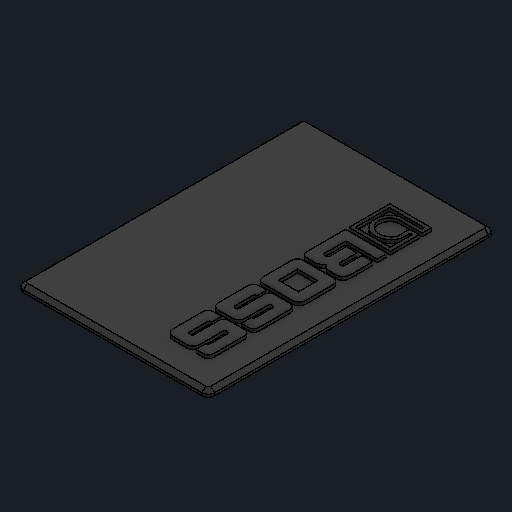
# Autodesk Inventor part: Pad
Saved by Autodesk Inventor 2026.2 (Build 302298000, 298)
## iProperties
Created: 2015-05-06
Part Number: Pad
Material: Rubber
Document SubType Name: Modeling
Designer: Philip
Density: 0.93 g/cm^3
Appearance: Rubber - Black
Author: Philip
Autodesk Inventor part; units mm, degrees
(part 1 of 2)
ref_plane "YZ Plane" through (0, 0, 0) normal (1, 0, 0) x (0, 1, 0)
ref_plane "XZ Plane" through (0, 0, 0) normal (0, 1, 0) x (-1, 0, 0)
ref_plane "XY Plane" through (0, 0, 0) normal (0, 0, 1) x (1, 0, 0)
sketch "Sketch1" plane through (0, 0, 0) normal (0, 1, 0) x (-1, 0, 0)
  line L0 (-19.05, 28.575) -> (19.05, 28.575)
  line L1 (19.05, 28.575) -> (19.05, -28.575)
  line L2 (19.05, -28.575) -> (-19.05, -28.575)
  line L3 (-19.05, -28.575) -> (-19.05, 28.575)
  point P0 (0, 0)
  dimension "d0" = 57.15
  dimension "d1" = 38.1
  dimension "d2" = 28.575
  dimension "d3" = 19.05
  constraints: 8 end point, 2 parallel, 1 horizontal, 1 perpendicular
  measures "d0" distance of L2.end L0.start
  measures "d1" distance of L1.end L2.end
  measures "d2" distance from line of L2 point (0, 0)
  measures "d3" distance from line of L1 point (0, 0)
extrude "Extrusion1" add sketch "Sketch1" along normal blind 1.27
fillet "Fillet1" radius 1.27 2 edges at (19.05, 0.635, 28.575) (-19.05, 0.635, 28.575)
fillet "Fillet1" radius 1.27 2 edges at (19.05, 0.635, -28.575) (-19.05, 0.635, -28.575)
chamfer "Chamfer1" distance 0.762 angle 45 8 edges at (19.05, 1.27, 0) (18.678, 1.27, -28.203) (0, 1.27, -28.575) (-18.678, 1.27, -28.203) (-19.05, 1.27, 0) (-18.678, 1.27, 28.203) (0, 1.27, 28.575) (18.678, 1.27, 28.203)
sketch "Sketch2" plane through (0, 1.27, 0) normal (0, 1, 0) x (1, 0, 0)
  spline S0 degree 3 poles (9.3958, 4.5889) (10.1252, 3.8936) (10.2655, 3.812) (10.8634, 3.789) (11.2905, 3.7727) (11.7187, 3.7634) (12.1459, 3.7736) (13.0489, 3.7954) (13.5879, 4.3543) (13.5894, 5.258) (13.5915, 6.5998) (13.5905, 7.9416) (13.5889, 9.2834) (13.5888, 9.4117) (13.575, 9.5399) (13.567, 9.6778) (12.8489, 9.6778) (12.163, 9.6778) (11.4348, 9.6778) (11.4348, 9.5086) (11.4348, 9.3648) (11.4348, 9.221) (11.4347, 8.2774) (11.4161, 7.3331) (11.443, 6.3902) (11.4552, 5.9625) (11.2394, 5.916) (10.901, 5.9027) (10.5127, 5.8874) (10.4743, 6.0999) (10.4779, 6.4041) (10.4876, 7.2297) (10.4812, 8.0555) (10.4812, 8.8813) (10.4812, 9.1406) (10.4812, 9.3999) (10.4812, 9.6605) (9.7415, 9.6605) (9.0682, 9.6605) (8.3475, 9.6605) (8.3475, 9.4797) (8.3475, 9.3219) (8.3475, 9.1641) (8.3475, 8.2647) (8.335, 7.3649) (8.3534, 6.4659) (8.3612, 6.0826) (8.2268, 5.9461) (7.8388, 5.9515) (7.4678, 5.9567) (7.305, 6.06) (7.3108, 6.4576) (7.3284, 7.6665) (7.3366, 8.8762) (7.307, 10.0846) (7.2961, 10.5311) (7.4609, 10.6266) (7.869, 10.6223) (9.594, 10.6041) (11.3193, 10.6146) (13.0445, 10.6146) (13.216, 10.6146) (13.3876, 10.6146) (13.5748, 10.6146) (13.5748, 11.2969) (13.5748, 11.9233) (13.5748, 12.5704) (10.8039, 12.5704) (8.0556, 12.5704) (5.2864, 12.5704) (5.2794, 12.4478) (5.2687, 12.3477) (5.2687, 12.2476) (5.2677, 9.8147) (5.2661, 7.3817) (5.2691, 4.9488) (5.27, 4.2597) (5.6025, 3.8797) (6.2966, 3.8167) (6.7503, 3.7755) (7.2103, 3.8092) (7.6658, 3.7819) (8.3846, 3.7388) (8.9658, 3.9758) (9.3958, 4.5889) knots 0 0 0 0 1 1 1 2 2 2 3 3 3 4 4 4 5 5 5 6 6 6 7 7 7 8 8 8 9 9 9 10 10 10 11 11 11 12 12 12 13 13 13 14 14 14 15 15 15 16 16 16 17 17 17 18 18 18 19 19 19 20 20 20 21 21 21 22 22 22 23 23 23 24 24 24 25 25 25 26 26 26 27 27 27 28 28 28 28
  line L0 (9.3958, 4.5889) -> (10.1252, 3.8936) construction
  line L1 (10.1252, 3.8936) -> (10.2655, 3.812) construction
  line L2 (10.2655, 3.812) -> (10.8634, 3.789) construction
  line L3 (10.8634, 3.789) -> (11.2905, 3.7727) construction
  line L4 (11.2905, 3.7727) -> (11.7187, 3.7634) construction
  line L5 (11.7187, 3.7634) -> (12.1459, 3.7736) construction
  line L6 (12.1459, 3.7736) -> (13.0489, 3.7954) construction
  line L7 (13.0489, 3.7954) -> (13.5879, 4.3543) construction
  line L8 (13.5879, 4.3543) -> (13.5894, 5.258) construction
  line L9 (13.5894, 5.258) -> (13.5915, 6.5998) construction
  line L10 (13.5915, 6.5998) -> (13.5905, 7.9416) construction
  line L11 (13.5905, 7.9416) -> (13.5889, 9.2834) construction
  line L12 (13.5889, 9.2834) -> (13.5888, 9.4117) construction
  line L13 (13.5888, 9.4117) -> (13.575, 9.5399) construction
  line L14 (13.575, 9.5399) -> (13.567, 9.6778) construction
  line L15 (13.567, 9.6778) -> (12.8489, 9.6778) construction
  line L16 (12.8489, 9.6778) -> (12.163, 9.6778) construction
  line L17 (12.163, 9.6778) -> (11.4348, 9.6778) construction
  line L18 (11.4348, 9.6778) -> (11.4348, 9.5086) construction
  line L19 (11.4348, 9.5086) -> (11.4348, 9.3648) construction
  line L20 (11.4348, 9.3648) -> (11.4348, 9.221) construction
  line L21 (11.4348, 9.221) -> (11.4347, 8.2774) construction
  line L22 (11.4347, 8.2774) -> (11.4161, 7.3331) construction
  line L23 (11.4161, 7.3331) -> (11.443, 6.3902) construction
  line L24 (11.443, 6.3902) -> (11.4552, 5.9625) construction
  line L25 (11.4552, 5.9625) -> (11.2394, 5.916) construction
  line L26 (11.2394, 5.916) -> (10.901, 5.9027) construction
  line L27 (10.901, 5.9027) -> (10.5127, 5.8874) construction
  line L28 (10.5127, 5.8874) -> (10.4743, 6.0999) construction
  line L29 (10.4743, 6.0999) -> (10.4779, 6.4041) construction
  line L30 (10.4779, 6.4041) -> (10.4876, 7.2297) construction
  line L31 (10.4876, 7.2297) -> (10.4812, 8.0555) construction
  line L32 (10.4812, 8.0555) -> (10.4812, 8.8813) construction
  line L33 (10.4812, 8.8813) -> (10.4812, 9.1406) construction
  line L34 (10.4812, 9.1406) -> (10.4812, 9.3999) construction
  line L35 (10.4812, 9.3999) -> (10.4812, 9.6605) construction
  line L36 (10.4812, 9.6605) -> (9.7415, 9.6605) construction
  line L37 (9.7415, 9.6605) -> (9.0682, 9.6605) construction
  line L38 (9.0682, 9.6605) -> (8.3475, 9.6605) construction
  line L39 (8.3475, 9.6605) -> (8.3475, 9.4797) construction
  line L40 (8.3475, 9.4797) -> (8.3475, 9.3219) construction
  line L41 (8.3475, 9.3219) -> (8.3475, 9.1641) construction
  line L42 (8.3475, 9.1641) -> (8.3475, 8.2647) construction
  line L43 (8.3475, 8.2647) -> (8.335, 7.3649) construction
  line L44 (8.335, 7.3649) -> (8.3534, 6.4659) construction
  line L45 (8.3534, 6.4659) -> (8.3612, 6.0826) construction
  line L46 (8.3612, 6.0826) -> (8.2268, 5.9461) construction
  line L47 (8.2268, 5.9461) -> (7.8388, 5.9515) construction
  line L48 (7.8388, 5.9515) -> (7.4678, 5.9567) construction
  line L49 (7.4678, 5.9567) -> (7.305, 6.06) construction
  line L50 (7.305, 6.06) -> (7.3108, 6.4576) construction
  line L51 (7.3108, 6.4576) -> (7.3284, 7.6665) construction
  line L52 (7.3284, 7.6665) -> (7.3366, 8.8762) construction
  line L53 (7.3366, 8.8762) -> (7.307, 10.0846) construction
  line L54 (7.307, 10.0846) -> (7.2961, 10.5311) construction
  line L55 (7.2961, 10.5311) -> (7.4609, 10.6266) construction
  line L56 (7.4609, 10.6266) -> (7.869, 10.6223) construction
  line L57 (7.869, 10.6223) -> (9.594, 10.6041) construction
  line L58 (9.594, 10.6041) -> (11.3193, 10.6146) construction
  line L59 (11.3193, 10.6146) -> (13.0445, 10.6146) construction
  line L60 (13.0445, 10.6146) -> (13.216, 10.6146) construction
  line L61 (13.216, 10.6146) -> (13.3876, 10.6146) construction
  line L62 (13.3876, 10.6146) -> (13.5748, 10.6146) construction
  line L63 (13.5748, 10.6146) -> (13.5748, 11.2969) construction
  line L64 (13.5748, 11.2969) -> (13.5748, 11.9233) construction
  line L65 (13.5748, 11.9233) -> (13.5748, 12.5704) construction
  line L66 (13.5748, 12.5704) -> (10.8039, 12.5704) construction
  line L67 (10.8039, 12.5704) -> (8.0556, 12.5704) construction
  line L68 (8.0556, 12.5704) -> (5.2864, 12.5704) construction
  line L69 (5.2864, 12.5704) -> (5.2794, 12.4478) construction
  line L70 (5.2794, 12.4478) -> (5.2687, 12.3477) construction
  line L71 (5.2687, 12.3477) -> (5.2687, 12.2476) construction
  line L72 (5.2687, 12.2476) -> (5.2677, 9.8147) construction
  line L73 (5.2677, 9.8147) -> (5.2661, 7.3817) construction
  line L74 (5.2661, 7.3817) -> (5.2691, 4.9488) construction
  line L75 (5.2691, 4.9488) -> (5.27, 4.2597) construction
  line L76 (5.27, 4.2597) -> (5.6025, 3.8797) construction
  line L77 (5.6025, 3.8797) -> (6.2966, 3.8167) construction
  line L78 (6.2966, 3.8167) -> (6.7503, 3.7755) construction
  line L79 (6.7503, 3.7755) -> (7.2103, 3.8092) construction
  line L80 (7.2103, 3.8092) -> (7.6658, 3.7819) construction
  line L81 (7.6658, 3.7819) -> (8.3846, 3.7388) construction
  line L82 (8.3846, 3.7388) -> (8.9658, 3.9758) construction
  line L83 (8.9658, 3.9758) -> (9.3958, 4.5889) construction
  spline S1 degree 3 poles (7.9431, -16.7748) (7.9431, -16.4138) (7.9431, -16.1057) (7.9431, -15.7977) (7.9431, -15.48) (7.9431, -15.1624) (7.9431, -14.8215) (7.4659, -14.8215) (7.0546, -14.8202) (6.6434, -14.8218) (5.6523, -14.8254) (5.2704, -15.1982) (5.2688, -16.1772) (5.2657, -18.0196) (5.266, -19.862) (5.2687, -21.7044) (5.27, -22.5866) (5.7744, -23.0965) (6.6665, -23.1073) (7.477, -23.1172) (8.2877, -23.1104) (9.0984, -23.1097) (10.1858, -23.1088) (10.6365, -22.667) (10.6389, -21.5905) (10.642, -20.1903) (10.6442, -18.79) (10.6364, -17.3899) (10.6347, -17.069) (10.6698, -16.8664) (11.0847, -16.8681) (11.5057, -16.8698) (11.5672, -17.0564) (11.5615, -17.4099) (11.5453, -18.4119) (11.5559, -19.4144) (11.5558, -20.4167) (11.5557, -20.6962) (11.6, -20.994) (11.2054, -21.0731) (11.1528, -21.0836) (11.089, -21.2069) (11.0878, -21.2789) (11.0783, -21.8651) (11.0824, -22.4515) (11.0824, -23.0807) (11.548, -23.0807) (11.9727, -23.0884) (12.397, -23.0791) (13.2638, -23.0602) (13.59, -22.7365) (13.5939, -21.8561) (13.6025, -19.9253) (13.6029, -17.9944) (13.5941, -16.0636) (13.5901, -15.2061) (13.1998, -14.8222) (12.349, -14.8143) (11.4648, -14.8061) (10.5803, -14.8113) (9.696, -14.8123) (8.6998, -14.8134) (8.3709, -15.1374) (8.3689, -16.1294) (8.366, -17.5886) (8.3607, -19.0479) (8.3735, -20.5069) (8.3766, -20.8568) (8.3246, -21.039) (7.8999, -21.0443) (7.4449, -21.0499) (7.4472, -20.8126) (7.4495, -20.4917) (7.4573, -19.4453) (7.4583, -18.3987) (7.4491, -17.3523) (7.4461, -17.01) (7.4589, -16.7084) (7.9431, -16.7748) knots 0 0 0 0 1 1 1 2 2 2 3 3 3 4 4 4 5 5 5 6 6 6 7 7 7 8 8 8 9 9 9 10 10 10 11 11 11 12 12 12 13 13 13 14 14 14 15 15 15 16 16 16 17 17 17 18 18 18 19 19 19 20 20 20 21 21 21 22 22 22 23 23 23 24 24 24 25 25 25 26 26 26 26
  line L84 (7.9431, -16.7748) -> (7.9431, -16.4138) construction
  line L85 (7.9431, -16.4138) -> (7.9431, -16.1057) construction
  line L86 (7.9431, -16.1057) -> (7.9431, -15.7977) construction
  line L87 (7.9431, -15.7977) -> (7.9431, -15.48) construction
  line L88 (7.9431, -15.48) -> (7.9431, -15.1624) construction
  line L89 (7.9431, -15.1624) -> (7.9431, -14.8215) construction
  line L90 (7.9431, -14.8215) -> (7.4659, -14.8215) construction
  line L91 (7.4659, -14.8215) -> (7.0546, -14.8202) construction
  line L92 (7.0546, -14.8202) -> (6.6434, -14.8218) construction
  line L93 (6.6434, -14.8218) -> (5.6523, -14.8254) construction
  line L94 (5.6523, -14.8254) -> (5.2704, -15.1982) construction
  line L95 (5.2704, -15.1982) -> (5.2688, -16.1772) construction
  line L96 (5.2688, -16.1772) -> (5.2657, -18.0196) construction
  line L97 (5.2657, -18.0196) -> (5.266, -19.862) construction
  line L98 (5.266, -19.862) -> (5.2687, -21.7044) construction
  line L99 (5.2687, -21.7044) -> (5.27, -22.5866) construction
  line L100 (5.27, -22.5866) -> (5.7744, -23.0965) construction
  line L101 (5.7744, -23.0965) -> (6.6665, -23.1073) construction
  line L102 (6.6665, -23.1073) -> (7.477, -23.1172) construction
  line L103 (7.477, -23.1172) -> (8.2877, -23.1104) construction
  line L104 (8.2877, -23.1104) -> (9.0984, -23.1097) construction
  line L105 (9.0984, -23.1097) -> (10.1858, -23.1088) construction
  line L106 (10.1858, -23.1088) -> (10.6365, -22.667) construction
  line L107 (10.6365, -22.667) -> (10.6389, -21.5905) construction
  line L108 (10.6389, -21.5905) -> (10.642, -20.1903) construction
  line L109 (10.642, -20.1903) -> (10.6442, -18.79) construction
  line L110 (10.6442, -18.79) -> (10.6364, -17.3899) construction
  line L111 (10.6364, -17.3899) -> (10.6347, -17.069) construction
  line L112 (10.6347, -17.069) -> (10.6698, -16.8664) construction
  line L113 (10.6698, -16.8664) -> (11.0847, -16.8681) construction
  line L114 (11.0847, -16.8681) -> (11.5057, -16.8698) construction
  line L115 (11.5057, -16.8698) -> (11.5672, -17.0564) construction
  line L116 (11.5672, -17.0564) -> (11.5615, -17.4099) construction
  line L117 (11.5615, -17.4099) -> (11.5453, -18.4119) construction
  line L118 (11.5453, -18.4119) -> (11.5559, -19.4144) construction
  line L119 (11.5559, -19.4144) -> (11.5558, -20.4167) construction
  line L120 (11.5558, -20.4167) -> (11.5557, -20.6962) construction
  line L121 (11.5557, -20.6962) -> (11.6, -20.994) construction
  line L122 (11.6, -20.994) -> (11.2054, -21.0731) construction
  line L123 (11.2054, -21.0731) -> (11.1528, -21.0836) construction
  line L124 (11.1528, -21.0836) -> (11.089, -21.2069) construction
  line L125 (11.089, -21.2069) -> (11.0878, -21.2789) construction
  line L126 (11.0878, -21.2789) -> (11.0783, -21.8651) construction
  line L127 (11.0783, -21.8651) -> (11.0824, -22.4515) construction
  line L128 (11.0824, -22.4515) -> (11.0824, -23.0807) construction
  line L129 (11.0824, -23.0807) -> (11.548, -23.0807) construction
  line L130 (11.548, -23.0807) -> (11.9727, -23.0884) construction
  line L131 (11.9727, -23.0884) -> (12.397, -23.0791) construction
  line L132 (12.397, -23.0791) -> (13.2638, -23.0602) construction
  line L133 (13.2638, -23.0602) -> (13.59, -22.7365) construction
  line L134 (13.59, -22.7365) -> (13.5939, -21.8561) construction
  line L135 (13.5939, -21.8561) -> (13.6025, -19.9253) construction
  line L136 (13.6025, -19.9253) -> (13.6029, -17.9944) construction
  line L137 (13.6029, -17.9944) -> (13.5941, -16.0636) construction
  line L138 (13.5941, -16.0636) -> (13.5901, -15.2061) construction
  line L139 (13.5901, -15.2061) -> (13.1998, -14.8222) construction
  line L140 (13.1998, -14.8222) -> (12.349, -14.8143) construction
  line L141 (12.349, -14.8143) -> (11.4648, -14.8061) construction
  line L142 (11.4648, -14.8061) -> (10.5803, -14.8113) construction
  line L143 (10.5803, -14.8113) -> (9.696, -14.8123) construction
  line L144 (9.696, -14.8123) -> (8.6998, -14.8134) construction
  line L145 (8.6998, -14.8134) -> (8.3709, -15.1374) construction
  line L146 (8.3709, -15.1374) -> (8.3689, -16.1294) construction
  line L147 (8.3689, -16.1294) -> (8.366, -17.5886) construction
  line L148 (8.366, -17.5886) -> (8.3607, -19.0479) construction
  line L149 (8.3607, -19.0479) -> (8.3735, -20.5069) construction
  line L150 (8.3735, -20.5069) -> (8.3766, -20.8568) construction
  line L151 (8.3766, -20.8568) -> (8.3246, -21.039) construction
  line L152 (8.3246, -21.039) -> (7.8999, -21.0443) construction
  line L153 (7.8999, -21.0443) -> (7.4449, -21.0499) construction
  line L154 (7.4449, -21.0499) -> (7.4472, -20.8126) construction
  line L155 (7.4472, -20.8126) -> (7.4495, -20.4917) construction
  line L156 (7.4495, -20.4917) -> (7.4573, -19.4453) construction
  line L157 (7.4573, -19.4453) -> (7.4583, -18.3987) construction
  line L158 (7.4583, -18.3987) -> (7.4491, -17.3523) construction
  line L159 (7.4491, -17.3523) -> (7.4461, -17.01) construction
  line L160 (7.4461, -17.01) -> (7.4589, -16.7084) construction
  line L161 (7.4589, -16.7084) -> (7.9431, -16.7748) construction
  spline S2 degree 3 poles (11.0982, -14.0424) (11.5176, -14.0424) (11.9126, -14.0444) (12.3075, -14.042) (13.2574, -14.0363) (13.5918, -13.714) (13.595, -12.7686) (13.6014, -10.8663) (13.6019, -8.9639) (13.5951, -7.0616) (13.5918, -6.1469) (13.2212, -5.7761) (12.3009, -5.7635) (11.4162, -5.7514) (10.5313, -5.7577) (9.6465, -5.7611) (8.7208, -5.7646) (8.3714, -6.1148) (8.3692, -7.0474) (8.3655, -8.5368) (8.3598, -10.0263) (8.374, -11.5156) (8.3775, -11.8755) (8.2691, -12.0057) (7.8937, -12.0083) (7.5216, -12.011) (7.4454, -11.8575) (7.4486, -11.5343) (7.4595, -10.4579) (7.4657, -9.3811) (7.4452, -8.3049) (7.4383, -7.9392) (7.5276, -7.7083) (7.9204, -7.7064) (7.9204, -7.0566) (7.9204, -6.4424) (7.9204, -5.7791) (7.4463, -5.7791) (6.9936, -5.772) (6.5411, -5.7806) (5.6631, -5.7973) (5.2726, -6.1849) (5.2699, -7.0586) (5.2641, -8.9462) (5.2648, -10.8338) (5.2694, -12.7214) (5.2714, -13.5244) (5.791, -14.0457) (6.5964, -14.054) (7.4369, -14.0626) (8.28, -14.0158) (9.1175, -14.0665) (10.1292, -14.1277) (10.6751, -13.4777) (10.6493, -12.5259) (10.6116, -11.1407) (10.6462, -9.7536) (10.6351, -8.3675) (10.6324, -8.0225) (10.6797, -7.8275) (11.1092, -7.8323) (11.5187, -7.8369) (11.564, -8.0209) (11.5602, -8.3493) (11.5483, -9.3667) (11.5484, -10.3844) (11.56, -11.4018) (11.5639, -11.7457) (11.53, -12.0308) (11.0982, -12.0358) (11.0982, -12.7117) (11.0982, -13.3563) (11.0982, -14.0424) knots 0 0 0 0 1 1 1 2 2 2 3 3 3 4 4 4 5 5 5 6 6 6 7 7 7 8 8 8 9 9 9 10 10 10 11 11 11 12 12 12 13 13 13 14 14 14 15 15 15 16 16 16 17 17 17 18 18 18 19 19 19 20 20 20 21 21 21 22 22 22 23 23 23 24 24 24 24
  line L162 (11.0982, -14.0424) -> (11.5176, -14.0424) construction
  line L163 (11.5176, -14.0424) -> (11.9126, -14.0444) construction
  line L164 (11.9126, -14.0444) -> (12.3075, -14.042) construction
  line L165 (12.3075, -14.042) -> (13.2574, -14.0363) construction
  line L166 (13.2574, -14.0363) -> (13.5918, -13.714) construction
  line L167 (13.5918, -13.714) -> (13.595, -12.7686) construction
  line L168 (13.595, -12.7686) -> (13.6014, -10.8663) construction
  line L169 (13.6014, -10.8663) -> (13.6019, -8.9639) construction
  line L170 (13.6019, -8.9639) -> (13.5951, -7.0616) construction
  line L171 (13.5951, -7.0616) -> (13.5918, -6.1469) construction
  line L172 (13.5918, -6.1469) -> (13.2212, -5.7761) construction
  line L173 (13.2212, -5.7761) -> (12.3009, -5.7635) construction
  line L174 (12.3009, -5.7635) -> (11.4162, -5.7514) construction
  line L175 (11.4162, -5.7514) -> (10.5313, -5.7577) construction
  line L176 (10.5313, -5.7577) -> (9.6465, -5.7611) construction
  line L177 (9.6465, -5.7611) -> (8.7208, -5.7646) construction
  line L178 (8.7208, -5.7646) -> (8.3714, -6.1148) construction
  line L179 (8.3714, -6.1148) -> (8.3692, -7.0474) construction
  line L180 (8.3692, -7.0474) -> (8.3655, -8.5368) construction
  line L181 (8.3655, -8.5368) -> (8.3598, -10.0263) construction
  line L182 (8.3598, -10.0263) -> (8.374, -11.5156) construction
  line L183 (8.374, -11.5156) -> (8.3775, -11.8755) construction
  line L184 (8.3775, -11.8755) -> (8.2691, -12.0057) construction
  line L185 (8.2691, -12.0057) -> (7.8937, -12.0083) construction
  line L186 (7.8937, -12.0083) -> (7.5216, -12.011) construction
  line L187 (7.5216, -12.011) -> (7.4454, -11.8575) construction
  line L188 (7.4454, -11.8575) -> (7.4486, -11.5343) construction
  line L189 (7.4486, -11.5343) -> (7.4595, -10.4579) construction
  line L190 (7.4595, -10.4579) -> (7.4657, -9.3811) construction
  line L191 (7.4657, -9.3811) -> (7.4452, -8.3049) construction
  line L192 (7.4452, -8.3049) -> (7.4383, -7.9392) construction
  line L193 (7.4383, -7.9392) -> (7.5276, -7.7083) construction
  line L194 (7.5276, -7.7083) -> (7.9204, -7.7064) construction
  line L195 (7.9204, -7.7064) -> (7.9204, -7.0566) construction
  line L196 (7.9204, -7.0566) -> (7.9204, -6.4424) construction
  line L197 (7.9204, -6.4424) -> (7.9204, -5.7791) construction
  line L198 (7.9204, -5.7791) -> (7.4463, -5.7791) construction
  line L199 (7.4463, -5.7791) -> (6.9936, -5.772) construction
  line L200 (6.9936, -5.772) -> (6.5411, -5.7806) construction
  line L201 (6.5411, -5.7806) -> (5.6631, -5.7973) construction
  line L202 (5.6631, -5.7973) -> (5.2726, -6.1849) construction
  line L203 (5.2726, -6.1849) -> (5.2699, -7.0586) construction
  line L204 (5.2699, -7.0586) -> (5.2641, -8.9462) construction
  line L205 (5.2641, -8.9462) -> (5.2648, -10.8338) construction
  line L206 (5.2648, -10.8338) -> (5.2694, -12.7214) construction
  line L207 (5.2694, -12.7214) -> (5.2714, -13.5244) construction
  line L208 (5.2714, -13.5244) -> (5.791, -14.0457) construction
  line L209 (5.791, -14.0457) -> (6.5964, -14.054) construction
  line L210 (6.5964, -14.054) -> (7.4369, -14.0626) construction
  line L211 (7.4369, -14.0626) -> (8.28, -14.0158) construction
  line L212 (8.28, -14.0158) -> (9.1175, -14.0665) construction
  line L213 (9.1175, -14.0665) -> (10.1292, -14.1277) construction
  line L214 (10.1292, -14.1277) -> (10.6751, -13.4777) construction
  line L215 (10.6751, -13.4777) -> (10.6493, -12.5259) construction
  line L216 (10.6493, -12.5259) -> (10.6116, -11.1407) construction
  line L217 (10.6116, -11.1407) -> (10.6462, -9.7536) construction
  line L218 (10.6462, -9.7536) -> (10.6351, -8.3675) construction
  line L219 (10.6351, -8.3675) -> (10.6324, -8.0225) construction
  line L220 (10.6324, -8.0225) -> (10.6797, -7.8275) construction
  line L221 (10.6797, -7.8275) -> (11.1092, -7.8323) construction
  line L222 (11.1092, -7.8323) -> (11.5187, -7.8369) construction
  line L223 (11.5187, -7.8369) -> (11.564, -8.0209) construction
  line L224 (11.564, -8.0209) -> (11.5602, -8.3493) construction
  line L225 (11.5602, -8.3493) -> (11.5483, -9.3667) construction
  line L226 (11.5483, -9.3667) -> (11.5484, -10.3844) construction
  line L227 (11.5484, -10.3844) -> (11.56, -11.4018) construction
  line L228 (11.56, -11.4018) -> (11.5639, -11.7457) construction
  line L229 (11.5639, -11.7457) -> (11.53, -12.0308) construction
  line L230 (11.53, -12.0308) -> (11.0982, -12.0358) construction
  line L231 (11.0982, -12.0358) -> (11.0982, -12.7117) construction
  line L232 (11.0982, -12.7117) -> (11.0982, -13.3563) construction
  line L233 (11.0982, -13.3563) -> (11.0982, -14.0424) construction
  spline S3 degree 3 poles (9.3804, 2.9807) (8.4379, 2.9807) (7.4953, 2.9896) (6.5529, 2.9781) (5.6541, 2.9672) (5.2718, 2.5752) (5.2694, 1.6722) (5.2646, -0.1097) (5.2646, -1.8916) (5.2693, -3.6735) (5.2717, -4.5581) (5.7101, -4.9936) (6.6079, -4.9965) (8.4634, -5.0026) (10.319, -5.0021) (12.1745, -4.9968) (13.0355, -4.9943) (13.5954, -4.4181) (13.5967, -3.5457) (13.5992, -1.8374) (13.5998, -0.1291) (13.5964, 1.5792) (13.5947, 2.4771) (13.1033, 2.9736) (12.2079, 2.9797) (11.2654, 2.9861) (10.3229, 2.9811) (9.3804, 2.9807) knots 0 0 0 0 1 1 1 2 2 2 3 3 3 4 4 4 5 5 5 6 6 6 7 7 7 8 8 8 9 9 9 9
  line L234 (9.3804, 2.9807) -> (8.4379, 2.9807) construction
  line L235 (8.4379, 2.9807) -> (7.4953, 2.9896) construction
  line L236 (7.4953, 2.9896) -> (6.5529, 2.9781) construction
  line L237 (6.5529, 2.9781) -> (5.6541, 2.9672) construction
  line L238 (5.6541, 2.9672) -> (5.2718, 2.5752) construction
  line L239 (5.2718, 2.5752) -> (5.2694, 1.6722) construction
  line L240 (5.2694, 1.6722) -> (5.2646, -0.1097) construction
  line L241 (5.2646, -0.1097) -> (5.2646, -1.8916) construction
  line L242 (5.2646, -1.8916) -> (5.2693, -3.6735) construction
  line L243 (5.2693, -3.6735) -> (5.2717, -4.5581) construction
  line L244 (5.2717, -4.5581) -> (5.7101, -4.9936) construction
  line L245 (5.7101, -4.9936) -> (6.6079, -4.9965) construction
  line L246 (6.6079, -4.9965) -> (8.4634, -5.0026) construction
  line L247 (8.4634, -5.0026) -> (10.319, -5.0021) construction
  line L248 (10.319, -5.0021) -> (12.1745, -4.9968) construction
  line L249 (12.1745, -4.9968) -> (13.0355, -4.9943) construction
  line L250 (13.0355, -4.9943) -> (13.5954, -4.4181) construction
  line L251 (13.5954, -4.4181) -> (13.5967, -3.5457) construction
  line L252 (13.5967, -3.5457) -> (13.5992, -1.8374) construction
  line L253 (13.5992, -1.8374) -> (13.5998, -0.1291) construction
  line L254 (13.5998, -0.1291) -> (13.5964, 1.5792) construction
  line L255 (13.5964, 1.5792) -> (13.5947, 2.4771) construction
  line L256 (13.5947, 2.4771) -> (13.1033, 2.9736) construction
  line L257 (13.1033, 2.9736) -> (12.2079, 2.9797) construction
  line L258 (12.2079, 2.9797) -> (11.2654, 2.9861) construction
  line L259 (11.2654, 2.9861) -> (10.3229, 2.9811) construction
  line L260 (10.3229, 2.9811) -> (9.3804, 2.9807) construction
  spline S4 degree 3 poles (13.5547, 21.4139) (10.7687, 21.4139) (8.0328, 21.4139) (5.2802, 21.4139) (5.2802, 18.6862) (5.2802, 15.9827) (5.2802, 13.2651) (8.0517, 13.2651) (10.7965, 13.2651) (13.5455, 13.2651) (13.5455, 15.191) (13.5455, 17.0836) (13.5455, 18.9818) (12.9033, 18.9818) (12.2921, 18.9818) (11.6488, 18.9818) (11.6488, 18.4267) (11.6155, 17.896) (11.6553, 17.3708) (11.7606, 15.9826) (10.723, 15.3515) (9.7967, 15.1936) (8.4636, 14.9664) (7.1726, 15.9402) (7.0798, 17.2739) (7.0047, 18.3535) (7.7939, 19.6173) (9.3599, 19.5716) (10.5968, 19.5355) (11.8356, 19.5635) (13.0735, 19.5654) (13.2295, 19.5656) (13.3856, 19.5794) (13.5547, 19.5876) (13.5547, 20.2145) (13.5547, 20.7978) (13.5547, 21.4139) knots 0 0 0 0 1 1 1 2 2 2 3 3 3 4 4 4 5 5 5 6 6 6 7 7 7 8 8 8 9 9 9 10 10 10 11 11 11 12 12 12 12
  line L261 (13.5547, 21.4139) -> (10.7687, 21.4139) construction
  line L262 (10.7687, 21.4139) -> (8.0328, 21.4139) construction
  line L263 (8.0328, 21.4139) -> (5.2802, 21.4139) construction
  line L264 (5.2802, 21.4139) -> (5.2802, 18.6862) construction
  line L265 (5.2802, 18.6862) -> (5.2802, 15.9827) construction
  line L266 (5.2802, 15.9827) -> (5.2802, 13.2651) construction
  line L267 (5.2802, 13.2651) -> (8.0517, 13.2651) construction
  line L268 (8.0517, 13.2651) -> (10.7965, 13.2651) construction
  line L269 (10.7965, 13.2651) -> (13.5455, 13.2651) construction
  line L270 (13.5455, 13.2651) -> (13.5455, 15.191) construction
  line L271 (13.5455, 15.191) -> (13.5455, 17.0836) construction
  line L272 (13.5455, 17.0836) -> (13.5455, 18.9818) construction
  line L273 (13.5455, 18.9818) -> (12.9033, 18.9818) construction
  line L274 (12.9033, 18.9818) -> (12.2921, 18.9818) construction
  line L275 (12.2921, 18.9818) -> (11.6488, 18.9818) construction
  line L276 (11.6488, 18.9818) -> (11.6488, 18.4267) construction
  line L277 (11.6488, 18.4267) -> (11.6155, 17.896) construction
  line L278 (11.6155, 17.896) -> (11.6553, 17.3708) construction
  line L279 (11.6553, 17.3708) -> (11.7606, 15.9826) construction
  line L280 (11.7606, 15.9826) -> (10.723, 15.3515) construction
  line L281 (10.723, 15.3515) -> (9.7967, 15.1936) construction
  line L282 (9.7967, 15.1936) -> (8.4636, 14.9664) construction
  line L283 (8.4636, 14.9664) -> (7.1726, 15.9402) construction
  line L284 (7.1726, 15.9402) -> (7.0798, 17.2739) construction
  line L285 (7.0798, 17.2739) -> (7.0047, 18.3535) construction
  line L286 (7.0047, 18.3535) -> (7.7939, 19.6173) construction
  line L287 (7.7939, 19.6173) -> (9.3599, 19.5716) construction
  line L288 (9.3599, 19.5716) -> (10.5968, 19.5355) construction
  line L289 (10.5968, 19.5355) -> (11.8356, 19.5635) construction
  line L290 (11.8356, 19.5635) -> (13.0735, 19.5654) construction
  line L291 (13.0735, 19.5654) -> (13.2295, 19.5656) construction
  line L292 (13.2295, 19.5656) -> (13.3856, 19.5794) construction
  line L293 (13.3856, 19.5794) -> (13.5547, 19.5876) construction
  line L294 (13.5547, 19.5876) -> (13.5547, 20.2145) construction
  line L295 (13.5547, 20.2145) -> (13.5547, 20.7978) construction
  line L296 (13.5547, 20.7978) -> (13.5547, 21.4139) construction
  spline S5 degree 3 poles (9.3958, 4.5889) (8.9658, 3.9758) (8.3846, 3.7388) (7.6658, 3.7819) (7.2103, 3.8092) (6.7503, 3.7755) (6.2966, 3.8167) (5.6025, 3.8797) (5.27, 4.2597) (5.2691, 4.9488) (5.2661, 7.3817) (5.2677, 9.8147) (5.2687, 12.2476) (5.2687, 12.3477) (5.2794, 12.4478) (5.2864, 12.5704) (8.0556, 12.5704) (10.8039, 12.5704) (13.5748, 12.5704) (13.5748, 11.9233) (13.5748, 11.2969) (13.5748, 10.6146) (13.3876, 10.6146) (13.216, 10.6146) (13.0445, 10.6146) (11.3193, 10.6146) (9.594, 10.6041) (7.869, 10.6223) (7.4609, 10.6266) (7.2961, 10.5311) (7.307, 10.0846) (7.3366, 8.8762) (7.3284, 7.6665) (7.3108, 6.4576) (7.305, 6.06) (7.4678, 5.9567) (7.8388, 5.9515) (8.2268, 5.9461) (8.3612, 6.0826) (8.3534, 6.4659) (8.335, 7.3649) (8.3475, 8.2647) (8.3475, 9.1641) (8.3475, 9.3219) (8.3475, 9.4797) (8.3475, 9.6605) (9.0682, 9.6605) (9.7415, 9.6605) (10.4812, 9.6605) (10.4812, 9.3999) (10.4812, 9.1406) (10.4812, 8.8813) (10.4812, 8.0555) (10.4876, 7.2297) (10.4779, 6.4041) (10.4743, 6.0999) (10.5127, 5.8874) (10.901, 5.9027) (11.2394, 5.916) (11.4552, 5.9625) (11.443, 6.3902) (11.4161, 7.3331) (11.4347, 8.2774) (11.4348, 9.221) (11.4348, 9.3648) (11.4348, 9.5086) (11.4348, 9.6778) (12.163, 9.6778) (12.8489, 9.6778) (13.567, 9.6778) (13.575, 9.5399) (13.5888, 9.4117) (13.5889, 9.2834) (13.5905, 7.9416) (13.5915, 6.5998) (13.5894, 5.258) (13.5879, 4.3543) (13.0489, 3.7954) (12.1459, 3.7736) (11.7187, 3.7634) (11.2905, 3.7727) (10.8634, 3.789) (10.2655, 3.812) (10.1252, 3.8936) (9.3958, 4.5889) knots 0 0 0 0 1 1 1 2 2 2 3 3 3 4 4 4 5 5 5 6 6 6 7 7 7 8 8 8 9 9 9 10 10 10 11 11 11 12 12 12 13 13 13 14 14 14 15 15 15 16 16 16 17 17 17 18 18 18 19 19 19 20 20 20 21 21 21 22 22 22 23 23 23 24 24 24 25 25 25 26 26 26 27 27 27 28 28 28 28
  line L297 (9.3958, 4.5889) -> (8.9658, 3.9758) construction
  line L298 (8.9658, 3.9758) -> (8.3846, 3.7388) construction
  line L299 (8.3846, 3.7388) -> (7.6658, 3.7819) construction
  line L300 (7.6658, 3.7819) -> (7.2103, 3.8092) construction
  line L301 (7.2103, 3.8092) -> (6.7503, 3.7755) construction
  line L302 (6.7503, 3.7755) -> (6.2966, 3.8167) construction
  line L303 (6.2966, 3.8167) -> (5.6025, 3.8797) construction
  line L304 (5.6025, 3.8797) -> (5.27, 4.2597) construction
  line L305 (5.27, 4.2597) -> (5.2691, 4.9488) construction
  line L306 (5.2691, 4.9488) -> (5.2661, 7.3817) construction
  line L307 (5.2661, 7.3817) -> (5.2677, 9.8147) construction
  line L308 (5.2677, 9.8147) -> (5.2687, 12.2476) construction
  line L309 (5.2687, 12.2476) -> (5.2687, 12.3477) construction
  line L310 (5.2687, 12.3477) -> (5.2794, 12.4478) construction
  line L311 (5.2794, 12.4478) -> (5.2864, 12.5704) construction
  line L312 (5.2864, 12.5704) -> (8.0556, 12.5704) construction
  line L313 (8.0556, 12.5704) -> (10.8039, 12.5704) construction
  line L314 (10.8039, 12.5704) -> (13.5748, 12.5704) construction
  line L315 (13.5748, 12.5704) -> (13.5748, 11.9233) construction
  line L316 (13.5748, 11.9233) -> (13.5748, 11.2969) construction
  line L317 (13.5748, 11.2969) -> (13.5748, 10.6146) construction
  line L318 (13.5748, 10.6146) -> (13.3876, 10.6146) construction
  line L319 (13.3876, 10.6146) -> (13.216, 10.6146) construction
  line L320 (13.216, 10.6146) -> (13.0445, 10.6146) construction
  line L321 (13.0445, 10.6146) -> (11.3193, 10.6146) construction
  line L322 (11.3193, 10.6146) -> (9.594, 10.6041) construction
  line L323 (9.594, 10.6041) -> (7.869, 10.6223) construction
  line L324 (7.869, 10.6223) -> (7.4609, 10.6266) construction
  line L325 (7.4609, 10.6266) -> (7.2961, 10.5311) construction
  line L326 (7.2961, 10.5311) -> (7.307, 10.0846) construction
  line L327 (7.307, 10.0846) -> (7.3366, 8.8762) construction
  line L328 (7.3366, 8.8762) -> (7.3284, 7.6665) construction
  line L329 (7.3284, 7.6665) -> (7.3108, 6.4576) construction
  line L330 (7.3108, 6.4576) -> (7.305, 6.06) construction
  line L331 (7.305, 6.06) -> (7.4678, 5.9567) construction
  line L332 (7.4678, 5.9567) -> (7.8388, 5.9515) construction
  line L333 (7.8388, 5.9515) -> (8.2268, 5.9461) construction
  line L334 (8.2268, 5.9461) -> (8.3612, 6.0826) construction
  line L335 (8.3612, 6.0826) -> (8.3534, 6.4659) construction
  line L336 (8.3534, 6.4659) -> (8.335, 7.3649) construction
  line L337 (8.335, 7.3649) -> (8.3475, 8.2647) construction
  line L338 (8.3475, 8.2647) -> (8.3475, 9.1641) construction
  line L339 (8.3475, 9.1641) -> (8.3475, 9.3219) construction
  line L340 (8.3475, 9.3219) -> (8.3475, 9.4797) construction
  line L341 (8.3475, 9.4797) -> (8.3475, 9.6605) construction
  line L342 (8.3475, 9.6605) -> (9.0682, 9.6605) construction
  line L343 (9.0682, 9.6605) -> (9.7415, 9.6605) construction
  line L344 (9.7415, 9.6605) -> (10.4812, 9.6605) construction
  line L345 (10.4812, 9.6605) -> (10.4812, 9.3999) construction
  line L346 (10.4812, 9.3999) -> (10.4812, 9.1406) construction
  line L347 (10.4812, 9.1406) -> (10.4812, 8.8813) construction
  line L348 (10.4812, 8.8813) -> (10.4812, 8.0555) construction
  line L349 (10.4812, 8.0555) -> (10.4876, 7.2297) construction
  line L350 (10.4876, 7.2297) -> (10.4779, 6.4041) construction
  line L351 (10.4779, 6.4041) -> (10.4743, 6.0999) construction
  line L352 (10.4743, 6.0999) -> (10.5127, 5.8874) construction
  line L353 (10.5127, 5.8874) -> (10.901, 5.9027) construction
  line L354 (10.901, 5.9027) -> (11.2394, 5.916) construction
  line L355 (11.2394, 5.916) -> (11.4552, 5.9625) construction
  line L356 (11.4552, 5.9625) -> (11.443, 6.3902) construction
  line L357 (11.443, 6.3902) -> (11.4161, 7.3331) construction
  line L358 (11.4161, 7.3331) -> (11.4347, 8.2774) construction
  line L359 (11.4347, 8.2774) -> (11.4348, 9.221) construction
  line L360 (11.4348, 9.221) -> (11.4348, 9.3648) construction
  line L361 (11.4348, 9.3648) -> (11.4348, 9.5086) construction
  line L362 (11.4348, 9.5086) -> (11.4348, 9.6778) construction
  line L363 (11.4348, 9.6778) -> (12.163, 9.6778) construction
  line L364 (12.163, 9.6778) -> (12.8489, 9.6778) construction
  line L365 (12.8489, 9.6778) -> (13.567, 9.6778) construction
  line L366 (13.567, 9.6778) -> (13.575, 9.5399) construction
  line L367 (13.575, 9.5399) -> (13.5888, 9.4117) construction
  line L368 (13.5888, 9.4117) -> (13.5889, 9.2834) construction
  line L369 (13.5889, 9.2834) -> (13.5905, 7.9416) construction
  line L370 (13.5905, 7.9416) -> (13.5915, 6.5998) construction
  line L371 (13.5915, 6.5998) -> (13.5894, 5.258) construction
  line L372 (13.5894, 5.258) -> (13.5879, 4.3543) construction
  line L373 (13.5879, 4.3543) -> (13.0489, 3.7954) construction
  line L374 (13.0489, 3.7954) -> (12.1459, 3.7736) construction
  line L375 (12.1459, 3.7736) -> (11.7187, 3.7634) construction
  line L376 (11.7187, 3.7634) -> (11.2905, 3.7727) construction
  line L377 (11.2905, 3.7727) -> (10.8634, 3.789) construction
  line L378 (10.8634, 3.789) -> (10.2655, 3.812) construction
  line L379 (10.2655, 3.812) -> (10.1252, 3.8936) construction
  line L380 (10.1252, 3.8936) -> (9.3958, 4.5889) construction
  spline S6 degree 3 poles (7.9431, -16.7748) (7.4589, -16.7084) (7.4461, -17.01) (7.4491, -17.3523) (7.4583, -18.3987) (7.4573, -19.4453) (7.4495, -20.4917) (7.4472, -20.8126) (7.4449, -21.0499) (7.8999, -21.0443) (8.3246, -21.039) (8.3766, -20.8568) (8.3735, -20.5069) (8.3607, -19.0479) (8.366, -17.5886) (8.3689, -16.1294) (8.3709, -15.1374) (8.6998, -14.8134) (9.696, -14.8123) (10.5803, -14.8113) (11.4648, -14.8061) (12.349, -14.8143) (13.1998, -14.8222) (13.5901, -15.2061) (13.5941, -16.0636) (13.6029, -17.9944) (13.6025, -19.9253) (13.5939, -21.8561) (13.59, -22.7365) (13.2638, -23.0602) (12.397, -23.0791) (11.9727, -23.0884) (11.548, -23.0807) (11.0824, -23.0807) (11.0824, -22.4515) (11.0783, -21.8651) (11.0878, -21.2789) (11.089, -21.2069) (11.1528, -21.0836) (11.2054, -21.0731) (11.6, -20.994) (11.5557, -20.6962) (11.5558, -20.4167) (11.5559, -19.4144) (11.5453, -18.4119) (11.5615, -17.4099) (11.5672, -17.0564) (11.5057, -16.8698) (11.0847, -16.8681) (10.6698, -16.8664) (10.6347, -17.069) (10.6364, -17.3899) (10.6442, -18.79) (10.642, -20.1903) (10.6389, -21.5905) (10.6365, -22.667) (10.1858, -23.1088) (9.0984, -23.1097) (8.2877, -23.1104) (7.477, -23.1172) (6.6665, -23.1073) (5.7744, -23.0965) (5.27, -22.5866) (5.2687, -21.7044) (5.266, -19.862) (5.2657, -18.0196) (5.2688, -16.1772) (5.2704, -15.1982) (5.6523, -14.8254) (6.6434, -14.8218) (7.0546, -14.8202) (7.4659, -14.8215) (7.9431, -14.8215) (7.9431, -15.1624) (7.9431, -15.48) (7.9431, -15.7977) (7.9431, -16.1057) (7.9431, -16.4138) (7.9431, -16.7748) knots 0 0 0 0 1 1 1 2 2 2 3 3 3 4 4 4 5 5 5 6 6 6 7 7 7 8 8 8 9 9 9 10 10 10 11 11 11 12 12 12 13 13 13 14 14 14 15 15 15 16 16 16 17 17 17 18 18 18 19 19 19 20 20 20 21 21 21 22 22 22 23 23 23 24 24 24 25 25 25 26 26 26 26
  line L381 (7.9431, -16.7748) -> (7.4589, -16.7084) construction
  line L382 (7.4589, -16.7084) -> (7.4461, -17.01) construction
  line L383 (7.4461, -17.01) -> (7.4491, -17.3523) construction
  line L384 (7.4491, -17.3523) -> (7.4583, -18.3987) construction
  line L385 (7.4583, -18.3987) -> (7.4573, -19.4453) construction
  line L386 (7.4573, -19.4453) -> (7.4495, -20.4917) construction
  line L387 (7.4495, -20.4917) -> (7.4472, -20.8126) construction
  line L388 (7.4472, -20.8126) -> (7.4449, -21.0499) construction
  line L389 (7.4449, -21.0499) -> (7.8999, -21.0443) construction
  line L390 (7.8999, -21.0443) -> (8.3246, -21.039) construction
  line L391 (8.3246, -21.039) -> (8.3766, -20.8568) construction
  line L392 (8.3766, -20.8568) -> (8.3735, -20.5069) construction
  line L393 (8.3735, -20.5069) -> (8.3607, -19.0479) construction
  line L394 (8.3607, -19.0479) -> (8.366, -17.5886) construction
  line L395 (8.366, -17.5886) -> (8.3689, -16.1294) construction
  line L396 (8.3689, -16.1294) -> (8.3709, -15.1374) construction
  line L397 (8.3709, -15.1374) -> (8.6998, -14.8134) construction
  line L398 (8.6998, -14.8134) -> (9.696, -14.8123) construction
  line L399 (9.696, -14.8123) -> (10.5803, -14.8113) construction
  line L400 (10.5803, -14.8113) -> (11.4648, -14.8061) construction
  line L401 (11.4648, -14.8061) -> (12.349, -14.8143) construction
  line L402 (12.349, -14.8143) -> (13.1998, -14.8222) construction
  line L403 (13.1998, -14.8222) -> (13.5901, -15.2061) construction
  line L404 (13.5901, -15.2061) -> (13.5941, -16.0636) construction
  line L405 (13.5941, -16.0636) -> (13.6029, -17.9944) construction
  line L406 (13.6029, -17.9944) -> (13.6025, -19.9253) construction
  line L407 (13.6025, -19.9253) -> (13.5939, -21.8561) construction
  line L408 (13.5939, -21.8561) -> (13.59, -22.7365) construction
  line L409 (13.59, -22.7365) -> (13.2638, -23.0602) construction
  line L410 (13.2638, -23.0602) -> (12.397, -23.0791) construction
  line L411 (12.397, -23.0791) -> (11.9727, -23.0884) construction
  line L412 (11.9727, -23.0884) -> (11.548, -23.0807) construction
  line L413 (11.548, -23.0807) -> (11.0824, -23.0807) construction
  line L414 (11.0824, -23.0807) -> (11.0824, -22.4515) construction
  line L415 (11.0824, -22.4515) -> (11.0783, -21.8651) construction
  line L416 (11.0783, -21.8651) -> (11.0878, -21.2789) construction
  line L417 (11.0878, -21.2789) -> (11.089, -21.2069) construction
  line L418 (11.089, -21.2069) -> (11.1528, -21.0836) construction
  line L419 (11.1528, -21.0836) -> (11.2054, -21.0731) construction
  line L420 (11.2054, -21.0731) -> (11.6, -20.994) construction
  line L421 (11.6, -20.994) -> (11.5557, -20.6962) construction
  line L422 (11.5557, -20.6962) -> (11.5558, -20.4167) construction
  line L423 (11.5558, -20.4167) -> (11.5559, -19.4144) construction
  line L424 (11.5559, -19.4144) -> (11.5453, -18.4119) construction
  line L425 (11.5453, -18.4119) -> (11.5615, -17.4099) construction
  line L426 (11.5615, -17.4099) -> (11.5672, -17.0564) construction
  line L427 (11.5672, -17.0564) -> (11.5057, -16.8698) construction
  line L428 (11.5057, -16.8698) -> (11.0847, -16.8681) construction
  line L429 (11.0847, -16.8681) -> (10.6698, -16.8664) construction
  line L430 (10.6698, -16.8664) -> (10.6347, -17.069) construction
  line L431 (10.6347, -17.069) -> (10.6364, -17.3899) construction
  line L432 (10.6364, -17.3899) -> (10.6442, -18.79) construction
  line L433 (10.6442, -18.79) -> (10.642, -20.1903) construction
  line L434 (10.642, -20.1903) -> (10.6389, -21.5905) construction
  line L435 (10.6389, -21.5905) -> (10.6365, -22.667) construction
  line L436 (10.6365, -22.667) -> (10.1858, -23.1088) construction
  line L437 (10.1858, -23.1088) -> (9.0984, -23.1097) construction
  line L438 (9.0984, -23.1097) -> (8.2877, -23.1104) construction
  line L439 (8.2877, -23.1104) -> (7.477, -23.1172) construction
  line L440 (7.477, -23.1172) -> (6.6665, -23.1073) construction
  line L441 (6.6665, -23.1073) -> (5.7744, -23.0965) construction
  line L442 (5.7744, -23.0965) -> (5.27, -22.5866) construction
  line L443 (5.27, -22.5866) -> (5.2687, -21.7044) construction
  line L444 (5.2687, -21.7044) -> (5.266, -19.862) construction
  line L445 (5.266, -19.862) -> (5.2657, -18.0196) construction
  line L446 (5.2657, -18.0196) -> (5.2688, -16.1772) construction
  line L447 (5.2688, -16.1772) -> (5.2704, -15.1982) construction
  line L448 (5.2704, -15.1982) -> (5.6523, -14.8254) construction
  line L449 (5.6523, -14.8254) -> (6.6434, -14.8218) construction
  line L450 (6.6434, -14.8218) -> (7.0546, -14.8202) construction
  line L451 (7.0546, -14.8202) -> (7.4659, -14.8215) construction
  line L452 (7.4659, -14.8215) -> (7.9431, -14.8215) construction
  line L453 (7.9431, -14.8215) -> (7.9431, -15.1624) construction
  line L454 (7.9431, -15.1624) -> (7.9431, -15.48) construction
  line L455 (7.9431, -15.48) -> (7.9431, -15.7977) construction
  line L456 (7.9431, -15.7977) -> (7.9431, -16.1057) construction
  line L457 (7.9431, -16.1057) -> (7.9431, -16.4138) construction
  line L458 (7.9431, -16.4138) -> (7.9431, -16.7748) construction
  spline S7 degree 3 poles (11.0982, -14.0424) (11.0982, -13.3563) (11.0982, -12.7117) (11.0982, -12.0358) (11.53, -12.0308) (11.5639, -11.7457) (11.56, -11.4018) (11.5484, -10.3844) (11.5483, -9.3667) (11.5602, -8.3493) (11.564, -8.0209) (11.5187, -7.8369) (11.1092, -7.8323) (10.6797, -7.8275) (10.6324, -8.0225) (10.6351, -8.3675) (10.6462, -9.7536) (10.6116, -11.1407) (10.6493, -12.5259) (10.6751, -13.4777) (10.1292, -14.1277) (9.1175, -14.0665) (8.28, -14.0158) (7.4369, -14.0626) (6.5964, -14.054) (5.791, -14.0457) (5.2714, -13.5244) (5.2694, -12.7214) (5.2648, -10.8338) (5.2641, -8.9462) (5.2699, -7.0586) (5.2726, -6.1849) (5.6631, -5.7973) (6.5411, -5.7806) (6.9936, -5.772) (7.4463, -5.7791) (7.9204, -5.7791) (7.9204, -6.4424) (7.9204, -7.0566) (7.9204, -7.7064) (7.5276, -7.7083) (7.4383, -7.9392) (7.4452, -8.3049) (7.4657, -9.3811) (7.4595, -10.4579) (7.4486, -11.5343) (7.4454, -11.8575) (7.5216, -12.011) (7.8937, -12.0083) (8.2691, -12.0057) (8.3775, -11.8755) (8.374, -11.5156) (8.3598, -10.0263) (8.3655, -8.5368) (8.3692, -7.0474) (8.3714, -6.1148) (8.7208, -5.7646) (9.6465, -5.7611) (10.5313, -5.7577) (11.4162, -5.7514) (12.3009, -5.7635) (13.2212, -5.7761) (13.5918, -6.1469) (13.5951, -7.0616) (13.6019, -8.9639) (13.6014, -10.8663) (13.595, -12.7686) (13.5918, -13.714) (13.2574, -14.0363) (12.3075, -14.042) (11.9126, -14.0444) (11.5176, -14.0424) (11.0982, -14.0424) knots 0 0 0 0 1 1 1 2 2 2 3 3 3 4 4 4 5 5 5 6 6 6 7 7 7 8 8 8 9 9 9 10 10 10 11 11 11 12 12 12 13 13 13 14 14 14 15 15 15 16 16 16 17 17 17 18 18 18 19 19 19 20 20 20 21 21 21 22 22 22 23 23 23 24 24 24 24
  line L459 (11.0982, -14.0424) -> (11.0982, -13.3563) construction
  line L460 (11.0982, -13.3563) -> (11.0982, -12.7117) construction
  line L461 (11.0982, -12.7117) -> (11.0982, -12.0358) construction
  line L462 (11.0982, -12.0358) -> (11.53, -12.0308) construction
  line L463 (11.53, -12.0308) -> (11.5639, -11.7457) construction
  line L464 (11.5639, -11.7457) -> (11.56, -11.4018) construction
  line L465 (11.56, -11.4018) -> (11.5484, -10.3844) construction
  line L466 (11.5484, -10.3844) -> (11.5483, -9.3667) construction
  line L467 (11.5483, -9.3667) -> (11.5602, -8.3493) construction
  line L468 (11.5602, -8.3493) -> (11.564, -8.0209) construction
  line L469 (11.564, -8.0209) -> (11.5187, -7.8369) construction
  line L470 (11.5187, -7.8369) -> (11.1092, -7.8323) construction
  line L471 (11.1092, -7.8323) -> (10.6797, -7.8275) construction
  line L472 (10.6797, -7.8275) -> (10.6324, -8.0225) construction
  line L473 (10.6324, -8.0225) -> (10.6351, -8.3675) construction
  line L474 (10.6351, -8.3675) -> (10.6462, -9.7536) construction
  line L475 (10.6462, -9.7536) -> (10.6116, -11.1407) construction
  line L476 (10.6116, -11.1407) -> (10.6493, -12.5259) construction
  line L477 (10.6493, -12.5259) -> (10.6751, -13.4777) construction
  line L478 (10.6751, -13.4777) -> (10.1292, -14.1277) construction
  line L479 (10.1292, -14.1277) -> (9.1175, -14.0665) construction
  line L480 (9.1175, -14.0665) -> (8.28, -14.0158) construction
  line L481 (8.28, -14.0158) -> (7.4369, -14.0626) construction
  line L482 (7.4369, -14.0626) -> (6.5964, -14.054) construction
  line L483 (6.5964, -14.054) -> (5.791, -14.0457) construction
  line L484 (5.791, -14.0457) -> (5.2714, -13.5244) construction
  line L485 (5.2714, -13.5244) -> (5.2694, -12.7214) construction
  line L486 (5.2694, -12.7214) -> (5.2648, -10.8338) construction
  line L487 (5.2648, -10.8338) -> (5.2641, -8.9462) construction
  line L488 (5.2641, -8.9462) -> (5.2699, -7.0586) construction
  line L489 (5.2699, -7.0586) -> (5.2726, -6.1849) construction
  line L490 (5.2726, -6.1849) -> (5.6631, -5.7973) construction
  line L491 (5.6631, -5.7973) -> (6.5411, -5.7806) construction
  line L492 (6.5411, -5.7806) -> (6.9936, -5.772) construction
  line L493 (6.9936, -5.772) -> (7.4463, -5.7791) construction
  line L494 (7.4463, -5.7791) -> (7.9204, -5.7791) construction
  line L495 (7.9204, -5.7791) -> (7.9204, -6.4424) construction
  line L496 (7.9204, -6.4424) -> (7.9204, -7.0566) construction
  line L497 (7.9204, -7.0566) -> (7.9204, -7.7064) construction
  line L498 (7.9204, -7.7064) -> (7.5276, -7.7083) construction
  line L499 (7.5276, -7.7083) -> (7.4383, -7.9392) construction
  line L500 (7.4383, -7.9392) -> (7.4452, -8.3049) construction
  line L501 (7.4452, -8.3049) -> (7.4657, -9.3811) construction
  line L502 (7.4657, -9.3811) -> (7.4595, -10.4579) construction
  line L503 (7.4595, -10.4579) -> (7.4486, -11.5343) construction
  line L504 (7.4486, -11.5343) -> (7.4454, -11.8575) construction
  line L505 (7.4454, -11.8575) -> (7.5216, -12.011) construction
  line L506 (7.5216, -12.011) -> (7.8937, -12.0083) construction
  line L507 (7.8937, -12.0083) -> (8.2691, -12.0057) construction
  line L508 (8.2691, -12.0057) -> (8.3775, -11.8755) construction
  line L509 (8.3775, -11.8755) -> (8.374, -11.5156) construction
  line L510 (8.374, -11.5156) -> (8.3598, -10.0263) construction
  line L511 (8.3598, -10.0263) -> (8.3655, -8.5368) construction
  line L512 (8.3655, -8.5368) -> (8.3692, -7.0474) construction
  line L513 (8.3692, -7.0474) -> (8.3714, -6.1148) construction
  line L514 (8.3714, -6.1148) -> (8.7208, -5.7646) construction
  line L515 (8.7208, -5.7646) -> (9.6465, -5.7611) construction
  line L516 (9.6465, -5.7611) -> (10.5313, -5.7577) construction
  line L517 (10.5313, -5.7577) -> (11.4162, -5.7514) construction
  line L518 (11.4162, -5.7514) -> (12.3009, -5.7635) construction
  line L519 (12.3009, -5.7635) -> (13.2212, -5.7761) construction
  line L520 (13.2212, -5.7761) -> (13.5918, -6.1469) construction
  line L521 (13.5918, -6.1469) -> (13.5951, -7.0616) construction
  line L522 (13.5951, -7.0616) -> (13.6019, -8.9639) construction
  line L523 (13.6019, -8.9639) -> (13.6014, -10.8663) construction
  line L524 (13.6014, -10.8663) -> (13.595, -12.7686) construction
  line L525 (13.595, -12.7686) -> (13.5918, -13.714) construction
  line L526 (13.5918, -13.714) -> (13.2574, -14.0363) construction
  line L527 (13.2574, -14.0363) -> (12.3075, -14.042) construction
  line L528 (12.3075, -14.042) -> (11.9126, -14.0444) construction
  line L529 (11.9126, -14.0444) -> (11.5176, -14.0424) construction
  line L530 (11.5176, -14.0424) -> (11.0982, -14.0424) construction
  spline S8 degree 3 poles (9.3804, 2.9809) (10.3229, 2.9811) (11.2654, 2.9861) (12.2079, 2.9797) (13.1033, 2.9736) (13.5947, 2.4771) (13.5964, 1.5792) (13.5998, -0.1291) (13.5992, -1.8374) (13.5967, -3.5457) (13.5954, -4.4181) (13.0355, -4.9943) (12.1745, -4.9968) (10.319, -5.0021) (8.4634, -5.0026) (6.6079, -4.9965) (5.7101, -4.9936) (5.2717, -4.5581) (5.2693, -3.6735) (5.2646, -1.8916) (5.2646, -0.1097) (5.2694, 1.6722) (5.2718, 2.5752) (5.6541, 2.9672) (6.5529, 2.9781) (7.4953, 2.9896) (8.4379, 2.9807) (9.3804, 2.9809) knots 0 0 0 0 1 1 1 2 2 2 3 3 3 4 4 4 5 5 5 6 6 6 7 7 7 8 8 8 9 9 9 9
  line L531 (9.3804, 2.9809) -> (10.3229, 2.9811) construction
  line L532 (10.3229, 2.9811) -> (11.2654, 2.9861) construction
  line L533 (11.2654, 2.9861) -> (12.2079, 2.9797) construction
  line L534 (12.2079, 2.9797) -> (13.1033, 2.9736) construction
  line L535 (13.1033, 2.9736) -> (13.5947, 2.4771) construction
  line L536 (13.5947, 2.4771) -> (13.5964, 1.5792) construction
  line L537 (13.5964, 1.5792) -> (13.5998, -0.1291) construction
  line L538 (13.5998, -0.1291) -> (13.5992, -1.8374) construction
  line L539 (13.5992, -1.8374) -> (13.5967, -3.5457) construction
  line L540 (13.5967, -3.5457) -> (13.5954, -4.4181) construction
  line L541 (13.5954, -4.4181) -> (13.0355, -4.9943) construction
  line L542 (13.0355, -4.9943) -> (12.1745, -4.9968) construction
  line L543 (12.1745, -4.9968) -> (10.319, -5.0021) construction
  line L544 (10.319, -5.0021) -> (8.4634, -5.0026) construction
  line L545 (8.4634, -5.0026) -> (6.6079, -4.9965) construction
  line L546 (6.6079, -4.9965) -> (5.7101, -4.9936) construction
  line L547 (5.7101, -4.9936) -> (5.2717, -4.5581) construction
  line L548 (5.2717, -4.5581) -> (5.2693, -3.6735) construction
  line L549 (5.2693, -3.6735) -> (5.2646, -1.8916) construction
  line L550 (5.2646, -1.8916) -> (5.2646, -0.1097) construction
  line L551 (5.2646, -0.1097) -> (5.2694, 1.6722) construction
  line L552 (5.2694, 1.6722) -> (5.2718, 2.5752) construction
  line L553 (5.2718, 2.5752) -> (5.6541, 2.9672) construction
  line L554 (5.6541, 2.9672) -> (6.5529, 2.9781) construction
  line L555 (6.5529, 2.9781) -> (7.4953, 2.9896) construction
  line L556 (7.4953, 2.9896) -> (8.4379, 2.9807) construction